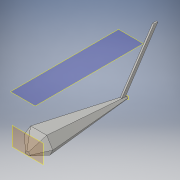
# Autodesk Inventor part: Buggy 2
Saved by Autodesk Inventor 2016 (Build 200138000, 138)
## iProperties
Created: 2016-04-13
Part Number: Buggy 2
Material: Generic
Document SubType Name: Modeling
Designer: rmarkowi
Density: 1 g/cm^3
Appearance: Default
Author: rmarkowi
Autodesk Inventor part; units mm, degrees
ref_plane "YZ Plane" through (0, 0, 0) normal (1, 0, 0) x (0, 1, 0)
ref_plane "XZ Plane" through (0, 0, 0) normal (0, 1, 0) x (-1, 0, 0)
sketch "Sketch1" plane through (0, 0, 0) normal (0, 0, 1) x (1, 0, 0)
  line L0 (0, 0) -> (39.3128, 0)
  line L1 (39.3128, 0) -> (49.1411, 19.6564)
  line L2 (49.1411, 19.6564) -> (28.1759, 54.1679)
  line L3 (0, 54.1679) -> (28.1759, 54.1679)
  line L4 (0, 54.1679) -> (0, 0) construction
  line L5 (0, 0) -> (-39.3128, 0)
  line L6 (-39.3128, 0) -> (-49.1411, 19.6564)
  line L7 (-49.1411, 19.6564) -> (-28.1759, 54.1679)
  line L8 (0, 54.1679) -> (-28.1759, 54.1679)
  constraints: 18 end point, 3 symmetric about line, 1 horizontal, 1 parallel, 1 vertical
ref_plane "Work Plane1" through (0, 0, -304.8) normal (0, 0, 1) x (1, 0, 0)
sketch "Sketch2" plane through (0, 0, -304.8) normal (0, 0, 1) x (1, 0, 0)
  line L0 (0, 0) -> (4.3244, 0)
  line L1 (4.3244, 0) -> (5.4055, 2.1622)
  line L2 (5.4055, 2.1622) -> (1.9294, 6.4866)
  line L3 (0, 6.4866) -> (1.9294, 6.4866)
  line L4 (0, 6.4866) -> (0, 0) construction
  line L5 (0, 0) -> (-4.3244, 0)
  line L6 (-4.3244, 0) -> (-5.4055, 2.1622)
  line L7 (-5.4055, 2.1622) -> (-1.9294, 6.4866)
  line L8 (0, 6.4866) -> (-1.9294, 6.4866)
  constraints: 18 end point, 4 symmetric about line, 2 point on line, 1 horizontal, 1 parallel, 1 vertical
ref_plane "Work Plane2" through (0, 0, 38.1) normal (0, 0, 1) x (1, 0, 0)
sketch "Sketch3" plane through (0, 0, 38.1) normal (0, 0, 1) x (1, 0, 0)
  line L0 (0, 0) -> (6.8628, 0)
  line L1 (6.8628, 0) -> (8.5786, 3.4314)
  line L2 (8.5786, 3.4314) -> (3.062, 10.2943)
  line L3 (0, 10.2943) -> (3.062, 10.2943)
  line L4 (0, 10.2943) -> (0, 0) construction
  line L5 (0, 0) -> (-6.8628, 0)
  line L6 (-6.8628, 0) -> (-8.5786, 3.4314)
  line L7 (-8.5786, 3.4314) -> (-3.062, 10.2943)
  line L8 (0, 10.2943) -> (-3.062, 10.2943)
  constraints: 18 end point, 4 symmetric about line, 2 point on line, 1 horizontal, 1 parallel, 1 vertical
loft "Loft1" add profiles "Sketch3", "Sketch1"
loft "Loft2" add profiles "Sketch1", "Sketch2"
sketch "Sketch4" plane through (-6.8628, 0, 38.1) normal (0, -1, 0) x (1, 0, 0)
  line L0 (11.1873, -342.9) -> (2.5384, -342.9) construction
  line L1 (6.8628, -342.9) -> (6.8628, 0) construction
  line L2 (6.8628, -332.5282) -> (9.525, -332.5282)
  line L3 (9.525, -332.5282) -> (9.525, -319.0875)
  line L4 (9.525, -319.0875) -> (6.8628, -319.0875)
  line L5 (6.8628, -332.5282) -> (4.2007, -332.5282)
  line L6 (4.2007, -332.5282) -> (4.2007, -319.0875)
  line L7 (4.2007, -319.0875) -> (6.8628, -319.0875)
  point P0 (6.8628, -38.1)
  constraints: 14 end point, 2 symmetric about line, 1 horizontal, 1 midpoint, 1 parallel, 1 perpendicular, 1 point on line, 1 vertical
ref_plane "Work Plane3" through (-6.8628, 177.8, 38.1) normal (0, -1, 0) x (1, 0, 0)
sketch "Sketch5" plane through (-6.8628, 177.8, 38.1) normal (0, -1, 0) x (1, 0, 0)
  line L0 (6.8628, -451.5907) -> (9.525, -451.5907)
  line L1 (9.525, -451.5907) -> (9.525, -438.15)
  line L2 (9.525, -438.15) -> (6.8628, -438.15)
  line L3 (6.8628, -451.5907) -> (4.2007, -451.5907)
  line L4 (4.2007, -451.5907) -> (4.2007, -438.15)
  line L5 (4.2007, -438.15) -> (6.8628, -438.15)
  line L6 (9.9248, 0) -> (3.8008, 0) construction
  line L7 (6.8628, 0) -> (6.8628, -342.9) construction
  point P0 (6.8628, -38.1)
  constraints: 14 end point, 1 horizontal, 1 midpoint, 1 parallel, 1 perpendicular, 1 vertical
loft "Loft3" add profiles "Sketch4", "Sketch5"
body "Solid1"
